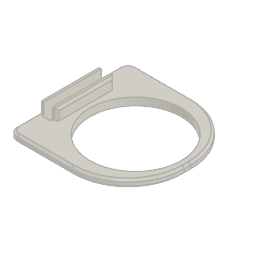
Hygrometer Bracket (Autodesk Fusion 360 design; units mm, degrees)
Autodesk Fusion 360 part; units mm, degrees
box "BoxPrimitive1" add length 55 width 55 height 3.5 placed x (0, 0, 1) y (0, -1, 0) z (1, 0, 0) at (0, 55, 0)
sketch "Body Features" plane through (0, 0, 0) normal (-1, 0, 0) x (0, -1, 0)
  line L0 (0, 55) -> (-55, 55)
  line L1 (-55, 55) -> (-55, 0)
  line L2 (-55, 0) -> (0, 0)
  line L3 (0, 0) -> (0, 55)
  line L4 (-27.5, 0) -> (-27.5, 55) construction
  circle A0 centre (-27.5, 31) radius 21
  line L5 (-40.75, 6) -> (-14.25, 6)
  line L6 (-14.25, 6) -> (-14.25, 2)
  line L7 (-14.25, 2) -> (-40.75, 2)
  line L8 (-40.75, 2) -> (-40.75, 6)
  line L9 (-40.75, 6) -> (-14.25, 2) construction
  line L10 (-14.25, 6) -> (-40.75, 2) construction
  line L11 (-14.25, 6) -> (-40.75, 6)
  line L12 (-40.75, 6) -> (-40.75, 8)
  line L13 (-40.75, 8) -> (-14.25, 8)
  line L14 (-14.25, 8) -> (-14.25, 6)
  line L15 (-40.75, 2) -> (-14.25, 2)
  line L16 (-14.25, 2) -> (-14.25, 0)
  line L17 (-14.25, 0) -> (-40.75, 0)
  line L18 (-40.75, 0) -> (-40.75, 2)
  point P0 (-27.5, 4)
  dimension "d8" = 42
  dimension "d9" = 24
  dimension "d11" = 2
  dimension "d12" = 4
  dimension "d22" = 26.5
  constraint midpoint L2 L4.start
  constraint midpoint L0 L4.end
  constraint coincident L4 A0.centre
  constraint horizontal L5
  constraint perpendicular L5 L6
  constraint parallel L5 L7
  constraint parallel L6 L8
  constraint coincident L9 P0
  constraint coincident L10 P0
  constraint coincident L4 P0
  constraint horizontal L11
  constraint vertical L12
  constraint horizontal L13
  constraint vertical L14
  constraint horizontal L15
  constraint vertical L16
  constraint horizontal L17
  constraint vertical L18
  constraint equal L14 L16
  constraint collinear L2 L17
  constraint collinear L8 L12
  constraint collinear L6 L16
  measures "d8" diameter of A0
  measures "d9" distance of L0 A0.centre
  measures "d11" distance of L6.end L16.end
  measures "d12" distance of L5.end L6.end
  measures "d22" distance of L5.end L5.start
extrude "Extrude1" add sketch "Body Features" along normal blind 5 contours L2 L7 L15 L16 L17 L18 | L5 L11 L12 L13 L14
extrude "Extrude2" cut sketch "Body Features" against normal blind 3.5 contours L5 L6 L7 L8 L11 L15 | A0
fillet "Fillet1" radius 26 2 edges at (1.75, 0, 55) (1.75, 55, 55)
chamfer "Chamfer1" distance 1 angle 45 2 edges at (0, 40.75, 4) (0, 14.25, 4)
fillet "Fillet2" radius 4 2 edges at (1.75, 55, 0) (1.75, 0, 0)
chamfer "Chamfer2" distance 1 angle 45 23 edges at (3.5, 0, 16.5) (3.5, 1.1716, 1.1716) (3.5, 27.5, 0) (3.5, 53.8284, 1.1716) (3.5, 55, 16.5) (3.5, 47.3848, 47.3848) (3.5, 27.5, 55) (3.5, 7.6152, 47.3848) (0, 0, 16.5) (0, 7.6152, 47.3848) (0, 27.5, 55) (0, 47.3848, 47.3848) (0, 55, 16.5) (0, 53.8284, 1.1716) (0, 45.875, 0) (0, 9.125, 0) (0, 1.1716, 1.1716) (-2.5, 14.25, 0) (-5, 27.5, 0) (-2.5, 40.75, 0) (-2.5, 14.25, 8) (-5, 27.5, 8) (-2.5, 40.75, 8)
sketch "Compliant mechanism" plane through (3.5, 0, 0) normal (1, 0, 0) x (0, 1, 0)
  line L0 (40.75, 6) -> (40.75, 2)
  line L1 (40.75, 2) -> (14.25, 2)
  line L2 (14.25, 2) -> (14.25, 6)
  line L3 (14.25, 6) -> (40.75, 6)
  circle A0 centre (27.5, 31) radius 21
  line L4 (1, 29) -> (1, 4)
  arc A1 (1, 4) -> (4, 1) centre (4, 4) ccw
  line L5 (4, 1) -> (51, 1)
  arc A2 (51, 1) -> (54, 4) centre (51, 4) ccw
  line L6 (54, 4) -> (54, 29)
  arc A3 (54, 29) -> (29, 54) centre (29, 29) ccw
  line L7 (29, 54) -> (26, 54)
  arc A4 (26, 54) -> (1, 29) centre (26, 29) ccw
  circle A5 centre (27.5, 31.35) radius 20.65 construction
  circle A6 centre (27.5, 31) radius 21
  line L8 (27.5, 31) -> (27.5, 52) construction
  circle A7 centre (27.5, 31.35) radius 22.5 construction
  line L9 (28.5, 10.9742) -> (28.4921, 10.5743) construction
  line L10 (28.5, 10.9742) -> (33.499, 10.8751)
  line L11 (28.4921, 10.5743) -> (32.0703, 10.5033)
  line L12 (27.5, 31) -> (27.5, -8.6192) construction
  line L13 (29.9639, 10.145) -> (32.0623, 10.1034)
  arc A8 (32.0623, 10.1034) -> (32.0703, 10.5033) centre (32.0663, 10.3034) ccw
  arc A9 (28.696, 10.9703) -> (28.696, 10.5703) centre (28.696, 10.7703) ccw
  line L14 (28.696, 10.5703) -> (28.696, 10.9703) construction
  point P0 (28.5, 10.7242)
  dimension "d24" = 41.3
  dimension "d26" = 45
  dimension "d27" = 0.4
  dimension "d28" = 5
  dimension "d29" = 1
  dimension "d30" = 0.25
  dimension "d31" = 0.4
  constraint coincident A0.centre A6.centre
  constraint coincident A0 L8.end
  constraint vertical L8
  constraint concentric A5 A7
  constraint coincident L8 A5.centre
  constraint coincident A5 L8.end
  constraint coincident A0 L10.end
  constraint perpendicular L9 L10
  constraint coincident A6 L11.end
  constraint parallel L10 L11
  constraint perpendicular L5 L12
  constraint coincident A5 P0
  constraint vertical L9.start P0
  constraint coincident A0 L13.start
  constraint parallel L11 L13
  constraint tangent L13 A8
  constraint coincident L11 A9.end
  constraint coincident L10 A9.start
  constraint tangent L9 A9
  constraint vertical L14
  constraint coincident A9.centre L14
  measures "d24" diameter of A5
  measures "d26" diameter of A7
  measures "d27" distance of L9.start L9.end
  measures "d28" distance of L9.start L10.end
  measures "d29" distance of L12 P0
  measures "d30" vertical distance of L9.start P0
  measures "d31" distance of L11 L13
extrude "Extrude3" [suppressed]
extrude "Extrude4" [suppressed]
ref_plane "WorkPlane1" through (1.75, 27.5, 16.5) normal (0, 1, 0) x (-1, 0, 0)
mirror "Mirror1" [suppressed]
move_body "Move1" bodies 1 to x (0, 0, -1) y (0, 1, 0) z (1, 0, 0) at (-27.5, -27.5, 4)
equation "d9 = d8 / 2 + 3 mm"
named bodies: "Hygrometer Bracket"
